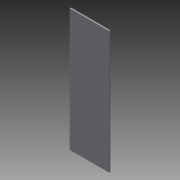
# Autodesk Inventor part: y-axis_mount_plate
Saved by Autodesk Inventor 2014 (Build 180170000, 170)
## iProperties
Created: 2014-08-18
Part Number: y-axis_mount_plate
Material: Generic
Document SubType Name: Modeling
Designer: Matthew
Density: 1 g/cm^3
Appearance: Default
Author: Matthew
Autodesk Inventor part; units mm, degrees
ref_plane "YZ Plane" through (0, 0, 0) normal (1, 0, 0) x (0, 1, 0)
ref_plane "XZ Plane" through (0, 0, 0) normal (0, 1, 0) x (-1, 0, 0)
ref_plane "XY Plane" through (0, 0, 0) normal (0, 0, 1) x (1, 0, 0)
sketch "Sketch1" plane through (0, 0, 0) normal (0, 1, 0) x (-1, 0, 0)
  line L0 (88.9, 276.0745) -> (-88.9, 276.0745)
  line L1 (-88.9, 276.0745) -> (-88.9, -276.0745)
  line L2 (-88.9, -276.0745) -> (88.9, -276.0745)
  line L3 (88.9, -276.0745) -> (88.9, 276.0745)
  line L4 (88.9, 276.0745) -> (-88.9, -276.0745) construction
  line L5 (-88.9, 276.0745) -> (88.9, -276.0745) construction
  point P0 (0, 0)
  dimension "d0" = 177.8
  dimension "d1" = 552.149
  constraints: 12 end point, 2 midpoint, 2 parallel, 1 horizontal, 1 perpendicular
  measures "d0" distance of L2.end L1.end
  measures "d1" distance of L0.end L1.end
extrude "Extrusion1" add sketch "Sketch1" along normal blind 6.35
body "Solid1"
